Autodesk Fusion 360 part; units mm, degrees
note: some values were not read from the file. Set by a fixed rule: which sketch regions a step uses.
(part 2 of 2)
sketch "Standoffs" plane through (0, 4, 0) normal (0, 1, 0) x (-1, 0, 0)
  line L0 (-79.851, -68.7474) -> (-79.851, -61.1474)
  line L1 (-79.851, -61.1474) -> (-69.251, -61.1474)
  line L2 (-69.251, -61.1474) -> (-69.251, -68.7474)
  line L3 (-69.251, -68.7474) -> (-79.851, -68.7474)
  line L4 (-70.751, -3.7474) -> (-70.751, -11.3474)
  line L5 (-70.751, -11.3474) -> (-78.351, -11.3474)
  line L6 (-78.351, -11.3474) -> (-78.351, -3.7474)
  line L7 (-78.351, -3.7474) -> (-70.751, -3.7474)
  line L8 (-78.351, 49.0551) -> (-78.351, 56.6551)
  line L9 (-78.351, 56.6551) -> (-70.751, 56.6551)
  line L10 (-70.751, 56.6551) -> (-70.751, 49.0551)
  line L11 (-70.751, 49.0551) -> (-78.351, 49.0551)
  line L12 (-70.751, 11.3526) -> (-70.751, 3.7526)
  line L13 (-70.751, 3.7526) -> (-78.351, 3.7526)
  line L14 (-78.351, 3.7526) -> (-78.351, 11.3526)
  line L15 (-78.351, 11.3526) -> (-70.751, 11.3526)
  line L16 (-79.851, -55.1474) -> (-79.851, -47.5474)
  line L17 (-79.851, -47.5474) -> (-69.251, -47.5474)
  line L18 (-69.251, -47.5474) -> (-69.251, -55.1474)
  line L19 (-69.251, -55.1474) -> (-79.851, -55.1474)
  line L20 (-70.751, -18.8474) -> (-70.751, -26.4474)
  line L21 (-70.751, -26.4474) -> (-78.351, -26.4474)
  line L22 (-78.351, -26.4474) -> (-78.351, -18.8474)
  line L23 (-78.351, -18.8474) -> (-70.751, -18.8474)
  line L24 (-78.351, 33.9551) -> (-78.351, 41.5551)
  line L25 (-78.351, 41.5551) -> (-70.751, 41.5551)
  line L26 (-70.751, 41.5551) -> (-70.751, 33.9551)
  line L27 (-70.751, 33.9551) -> (-78.351, 33.9551)
  line L28 (-70.751, 26.4526) -> (-70.751, 18.8526)
  line L29 (-70.751, 18.8526) -> (-78.351, 18.8526)
  line L30 (-78.351, 18.8526) -> (-78.351, 26.4526)
  line L31 (-78.351, 26.4526) -> (-70.751, 26.4526)
  line L32 (-78.351, -41.5474) -> (-78.351, -33.9474)
  line L33 (-78.351, -33.9474) -> (-70.751, -33.9474)
  line L34 (-70.751, -33.9474) -> (-70.751, -41.5474)
  line L35 (-70.751, -41.5474) -> (-78.351, -41.5474)
  line L36 (-81.051, -86.395) -> (-68.051, -86.395)
  line L37 (-68.051, -86.395) -> (-68.051, 62.605)
  line L38 (-68.051, 62.605) -> (-81.051, 62.605)
  line L39 (-81.051, 62.605) -> (-81.051, -86.395)
  line L40 (-81.051, -42.5474) -> (-68.051, -42.5474)
  line L41 (-68.051, -42.5474) -> (-68.051, -46.5474)
  line L42 (-68.051, -46.5474) -> (-81.051, -46.5474)
  line L43 (-81.051, -46.5474) -> (-81.051, -42.5474)
  line L44 (-68.051, -56.1474) -> (-81.051, -56.1474)
  line L45 (-81.051, -56.1474) -> (-81.051, -60.1474)
  line L46 (-81.051, -60.1474) -> (-68.051, -60.1474)
  line L47 (-68.051, -60.1474) -> (-68.051, -56.1474)
  line L48 (-68.051, -69.7474) -> (-81.051, -69.7474)
  line L49 (-81.051, -69.7474) -> (-81.051, -74.7474)
  line L50 (-81.051, -74.7474) -> (-68.051, -74.7474)
  line L51 (-68.051, -74.7474) -> (-68.051, -69.7474)
  line L52 (-68.051, -32.9474) -> (-81.051, -32.9474)
  line L53 (-81.051, -32.9474) -> (-81.051, -27.4474)
  line L54 (-81.051, -27.4474) -> (-68.051, -27.4474)
  line L55 (-68.051, -27.4474) -> (-68.051, -32.9474)
  line L56 (-68.051, -17.8474) -> (-81.051, -17.8474)
  line L57 (-81.051, -17.8474) -> (-81.051, -12.3474)
  line L58 (-81.051, -12.3474) -> (-68.051, -12.3474)
  line L59 (-68.051, -12.3474) -> (-68.051, -17.8474)
  line L60 (-68.051, -2.7474) -> (-81.051, -2.7474)
  line L61 (-81.051, -2.7474) -> (-81.051, 2.7526)
  line L62 (-81.051, 2.7526) -> (-68.051, 2.7526)
  line L63 (-68.051, 2.7526) -> (-68.051, -2.7474)
  line L64 (-68.051, 12.3526) -> (-81.051, 12.3526)
  line L65 (-81.051, 12.3526) -> (-81.051, 17.8526)
  line L66 (-81.051, 17.8526) -> (-68.051, 17.8526)
  line L67 (-68.051, 17.8526) -> (-68.051, 12.3526)
  line L68 (-68.051, 27.4526) -> (-81.051, 27.4526)
  line L69 (-81.051, 27.4526) -> (-81.051, 32.9551)
  line L70 (-81.051, 32.9551) -> (-68.051, 32.9551)
  line L71 (-68.051, 32.9551) -> (-68.051, 27.4526)
  line L72 (-68.051, 42.5551) -> (-81.051, 42.5551)
  line L73 (-81.051, 42.5551) -> (-81.051, 48.0551)
  line L74 (-81.051, 48.0551) -> (-68.051, 48.0551)
  line L75 (-68.051, 48.0551) -> (-68.051, 42.5551)
  line L76 (-68.051, 57.6551) -> (-81.051, 57.6551)
  line L77 (-81.051, 57.6551) -> (-81.051, 62.605)
  line L78 (-81.051, 62.605) -> (-68.051, 62.605)
  line L79 (-68.051, 62.605) -> (-68.051, 57.6551)
  line L80 (-32.451, 96.755) -> (-27.151, 96.755)
  line L81 (-27.151, 96.755) -> (-27.151, 86.755)
  line L82 (-27.151, 86.755) -> (-32.451, 86.755)
  line L83 (-32.451, 86.755) -> (-32.451, 96.755)
  line L84 (-17.551, 96.755) -> (-12.251, 96.755)
  line L85 (-12.251, 96.755) -> (-12.251, 86.755)
  line L86 (-12.251, 86.755) -> (-17.551, 86.755)
  line L87 (-17.551, 86.755) -> (-17.551, 96.755)
  line L88 (-2.651, 96.755) -> (2.649, 96.755)
  line L89 (2.649, 96.755) -> (2.649, 86.755)
  line L90 (2.649, 86.755) -> (-2.651, 86.755)
  line L91 (-2.651, 86.755) -> (-2.651, 96.755)
  line L92 (12.249, 96.755) -> (17.549, 96.755)
  line L93 (17.549, 96.755) -> (17.549, 86.755)
  line L94 (17.549, 86.755) -> (12.249, 86.755)
  line L95 (12.249, 86.755) -> (12.249, 96.755)
  line L96 (27.149, 96.755) -> (32.451, 96.755)
  line L97 (32.451, 96.755) -> (32.451, 86.755)
  line L98 (32.451, 86.755) -> (27.149, 86.755)
  line L99 (27.149, 86.755) -> (27.149, 96.755)
  line L100 (68, 42.5551) -> (81, 42.5551)
  line L101 (81, 42.5551) -> (81, 47.5551)
  line L102 (81, 47.5551) -> (68, 47.5551)
  line L103 (68, 47.5551) -> (68, 42.5551)
  line L104 (81, 32.9551) -> (68, 32.9551)
  line L105 (68, 32.9551) -> (68, 27.4526)
  line L106 (68, 27.4526) -> (81, 27.4526)
  line L107 (81, 27.4526) -> (81, 32.9551)
  line L108 (81, 17.8526) -> (68, 17.8526)
  line L109 (68, 17.8526) -> (68, 12.3526)
  line L110 (68, 12.3526) -> (81, 12.3526)
  line L111 (81, 12.3526) -> (81, 17.8526)
  line L112 (68, 2.7526) -> (81, 2.7526)
  line L113 (81, 2.7526) -> (81, -2.7474)
  line L114 (81, -2.7474) -> (68, -2.7474)
  line L115 (68, -2.7474) -> (68, 2.7526)
  line L116 (81, -12.3474) -> (68, -12.3474)
  line L117 (68, -12.3474) -> (68, -17.8474)
  line L118 (68, -17.8474) -> (81, -17.8474)
  line L119 (81, -17.8474) -> (81, -12.3474)
  line L120 (81, -27.4474) -> (68, -27.4474)
  line L121 (68, -27.4474) -> (68, -32.9474)
  line L122 (68, -32.9474) -> (81, -32.9474)
  line L123 (81, -32.9474) -> (81, -27.4474)
  line L124 (81, -42.5474) -> (68, -42.5474)
  line L125 (68, -42.5474) -> (68, -46.5474)
  line L126 (68, -46.5474) -> (81, -46.5474)
  line L127 (81, -46.5474) -> (81, -42.5474)
  line L128 (81, -56.1474) -> (68, -56.1474)
  line L129 (68, -56.1474) -> (68, -60.1474)
  line L130 (68, -60.1474) -> (81, -60.1474)
  line L131 (81, -60.1474) -> (81, -56.1474)
  line L132 (81, -69.7474) -> (68, -69.7474)
  line L133 (68, -69.7474) -> (68, -74.7474)
  line L134 (68, -74.7474) -> (81, -74.7474)
  line L135 (81, -74.7474) -> (81, -69.7474)
  line L136 (42.051, -86.755) -> (46.051, -86.755)
  line L137 (46.051, -86.755) -> (46.051, -96.755)
  line L138 (46.051, -96.755) -> (42.051, -96.755)
  line L139 (42.051, -96.755) -> (42.051, -86.755)
  line L140 (27.149, -86.755) -> (32.451, -86.755)
  line L141 (32.451, -86.755) -> (32.451, -96.755)
  line L142 (32.451, -96.755) -> (27.149, -96.755)
  line L143 (27.149, -96.755) -> (27.149, -86.755)
  line L144 (12.249, -86.755) -> (17.549, -86.755)
  line L145 (17.549, -86.755) -> (17.549, -96.755)
  line L146 (17.549, -96.755) -> (12.249, -96.755)
  line L147 (12.249, -96.755) -> (12.249, -86.755)
  line L148 (-2.651, -86.755) -> (2.649, -86.755)
  line L149 (2.649, -86.755) -> (2.649, -96.755)
  line L150 (2.649, -96.755) -> (-2.651, -96.755)
  line L151 (-2.651, -96.755) -> (-2.651, -86.755)
  line L152 (-17.551, -86.755) -> (-12.251, -86.755)
  line L153 (-12.251, -86.755) -> (-12.251, -96.755)
  line L154 (-12.251, -96.755) -> (-17.551, -96.755)
  line L155 (-17.551, -96.755) -> (-17.551, -86.755)
  line L156 (-32.451, -86.755) -> (-27.151, -86.755)
  line L157 (-27.151, -86.755) -> (-27.151, -96.755)
  line L158 (-27.151, -96.755) -> (-32.451, -96.755)
  line L159 (-32.451, -96.755) -> (-32.451, -86.755)
  line L160 (-46.051, -86.755) -> (-42.051, -86.755)
  line L161 (-42.051, -86.755) -> (-42.051, -96.755)
  line L162 (-42.051, -96.755) -> (-46.051, -96.755)
  line L163 (-46.051, -96.755) -> (-46.051, -86.755)
  line L164 (-33.451, 95.555) -> (-33.451, 87.955)
  line L165 (-26.151, 87.955) -> (-26.151, 95.555)
  line L166 (42.499, 86.755) -> (-42.501, 86.755)
  line L167 (-42.501, 96.755) -> (42.499, 96.755)
  line L168 (18.549, 87.955) -> (18.549, 95.555)
  line L169 (11.249, 95.555) -> (11.249, 87.955)
  line L170 (3.649, 87.955) -> (3.649, 95.555)
  line L171 (-3.651, 95.555) -> (-3.651, 87.955)
  line L172 (-18.551, 95.555) -> (-18.551, 87.955)
  line L173 (-11.251, 87.955) -> (-11.251, 95.555)
  line L174 (26.149, 95.555) -> (26.149, 87.955)
  line L175 (33.451, 87.955) -> (33.451, 95.555)
  line L176 (70.751, 41.5551) -> (78.351, 41.5551)
  line L177 (70.751, 26.4526) -> (78.351, 26.4526)
  line L178 (78.351, 33.9551) -> (70.751, 33.9551)
  line L179 (78.351, 18.8526) -> (70.751, 18.8526)
  line L180 (70.751, 11.3526) -> (78.351, 11.3526)
  line L181 (78.351, 3.7526) -> (70.751, 3.7526)
  line L182 (70.751, -3.7474) -> (78.351, -3.7474)
  line L183 (78.351, -11.3474) -> (70.751, -11.3474)
  line L184 (70.751, -18.8474) -> (78.351, -18.8474)
  line L185 (78.351, -26.4474) -> (70.751, -26.4474)
  line L186 (70.751, -33.9474) -> (78.351, -33.9474)
  line L187 (78.351, -41.5474) -> (70.751, -41.5474)
  line L188 (69.251, -47.5474) -> (79.851, -47.5474)
  line L189 (79.851, -55.1474) -> (69.251, -55.1474)
  line L190 (69.251, -61.1474) -> (79.851, -61.1474)
  line L191 (79.851, -68.7474) -> (69.251, -68.7474)
  line L192 (-58.499, -86.755) -> (58.501, -86.755)
  line L193 (58.501, -96.755) -> (-58.499, -96.755)
  line L194 (47.051, -95.555) -> (47.051, -87.955)
  line L195 (41.051, -87.955) -> (41.051, -95.555)
  line L196 (33.451, -95.555) -> (33.451, -87.955)
  line L197 (26.149, -87.955) -> (26.149, -95.555)
  line L198 (18.549, -95.555) -> (18.549, -87.955)
  line L199 (11.249, -87.955) -> (11.249, -95.555)
  line L200 (-47.051, -87.955) -> (-47.051, -95.555)
  line L201 (-41.051, -95.555) -> (-41.051, -87.955)
  line L202 (-33.451, -87.955) -> (-33.451, -95.555)
  line L203 (-26.151, -95.555) -> (-26.151, -87.955)
  line L204 (-18.551, -87.955) -> (-18.551, -95.555)
  line L205 (-11.251, -95.555) -> (-11.251, -87.955)
  line L206 (-3.651, -87.955) -> (-3.651, -95.555)
  line L207 (3.649, -95.555) -> (3.649, -87.955)
  dimension "d304" = 1
  dimension "d305" = 5
  dimension "d306" = 1
  dimension "d307" = 1
  dimension "d308" = 1.2
  dimension "d309" = 1
  dimension "d310" = 1
  dimension "d311" = 1
  dimension "d312" = 1
  dimension "d313" = 1
  dimension "d314" = 1
  dimension "d315" = 1
  dimension "d316" = 1
  dimension "d317" = 1
  dimension "d318" = 1
  dimension "d319" = 1
  dimension "d320" = 1
  dimension "d321" = 1
  dimension "d322" = 1
  dimension "d323" = 1
  dimension "d324" = 1
  dimension "d325" = 1
  dimension "d326" = 1
  dimension "d327" = 1
  dimension "d328" = 1
  dimension "d329" = 1
  dimension "d330" = 1
  dimension "d331" = 1
  dimension "d332" = 7.6
  dimension "d333" = 1
  dimension "d334" = 1
  dimension "d335" = 1
  dimension "d336" = 5
  dimension "d337" = 1
  dimension "d338" = 1
  dimension "d339" = 1
  dimension "d340" = 1
  dimension "d341" = 1
  dimension "d342" = 1
  dimension "d343" = 1
  dimension "d344" = 1
  dimension "d345" = 1
  dimension "d346" = 1
  dimension "d347" = 5.5
  dimension "d348" = 1
  dimension "d349" = 1
  dimension "d350" = 1
  dimension "d351" = 1
  dimension "d352" = 1
  dimension "d353" = 5
  dimension "d354" = 1
  dimension "d355" = 1
  dimension "d356" = 1
  dimension "d357" = 1
  dimension "d358" = 1
  dimension "d359" = 1
  dimension "d360" = 1
  dimension "d361" = 1
  dimension "d362" = 1
  dimension "d363" = 1
  dimension "d364" = 1
  dimension "d365" = 1
  dimension "d366" = 1
  dimension "d367" = 1
  constraint horizontal L40
  constraint vertical L41
  constraint horizontal L42
  constraint vertical L43
  constraint coincident L37 L41.end
  constraint coincident L39 L40.start
  constraint horizontal L44
  constraint vertical L45
  constraint horizontal L46
  constraint vertical L47
  constraint coincident L39 L45.end
  constraint coincident L37 L44.start
  constraint horizontal L48
  constraint vertical L49
  constraint horizontal L50
  constraint vertical L51
  constraint coincident L39 L49.end
  constraint coincident L37 L48.start
  constraint horizontal L52
  constraint vertical L53
  constraint horizontal L54
  constraint vertical L55
  constraint coincident L39 L53.end
  constraint coincident L37 L52.start
  constraint horizontal L56
  constraint vertical L57
  constraint horizontal L58
  constraint vertical L59
  constraint coincident L37 L56.start
  constraint horizontal L60
  constraint vertical L61
  constraint horizontal L62
  constraint vertical L63
  constraint coincident L39 L61.end
  constraint coincident L37 L60.start
  constraint horizontal L64
  constraint vertical L65
  constraint horizontal L66
  constraint vertical L67
  constraint coincident L39 L65.end
  constraint coincident L37 L64.start
  constraint horizontal L68
  constraint vertical L69
  constraint horizontal L70
  constraint vertical L71
  constraint coincident L39 L69.end
  constraint coincident L37 L68.start
  constraint horizontal L72
  constraint vertical L73
  constraint horizontal L74
  constraint vertical L75
  constraint coincident L39 L73.end
  constraint coincident L37 L72.start
  constraint horizontal L76
  constraint vertical L77
  constraint horizontal L78
  constraint vertical L79
  constraint coincident L38.end L39.start
  constraint coincident L37 L76.start
  constraint horizontal L80
  constraint vertical L81
  constraint horizontal L82
  constraint vertical L83
  constraint horizontal L84
  constraint vertical L85
  constraint horizontal L86
  constraint vertical L87
  constraint horizontal L88
  constraint vertical L89
  constraint horizontal L90
  constraint vertical L91
  constraint horizontal L92
  constraint vertical L93
  constraint horizontal L94
  constraint vertical L95
  constraint horizontal L96
  constraint vertical L97
  constraint horizontal L98
  constraint vertical L99
  constraint horizontal L100
  constraint vertical L101
  constraint horizontal L102
  constraint vertical L103
  constraint horizontal L104
  constraint vertical L105
  constraint horizontal L106
  constraint vertical L107
  constraint horizontal L108
  constraint vertical L109
  constraint horizontal L110
  constraint vertical L111
  constraint horizontal L112
  constraint vertical L113
  constraint horizontal L114
  constraint vertical L115
  constraint horizontal L116
  constraint vertical L117
  constraint horizontal L118
  constraint vertical L119
  constraint horizontal L120
  constraint vertical L121
  constraint horizontal L122
  constraint vertical L123
  constraint horizontal L124
  constraint vertical L125
  constraint horizontal L126
  constraint vertical L127
  constraint horizontal L128
  constraint vertical L129
  constraint horizontal L130
  constraint vertical L131
  constraint horizontal L132
  constraint vertical L133
  constraint horizontal L134
  constraint vertical L135
  constraint horizontal L136
  constraint vertical L137
  constraint horizontal L138
  constraint vertical L139
  constraint horizontal L140
  constraint vertical L141
  constraint horizontal L142
  constraint vertical L143
  constraint horizontal L144
  constraint vertical L145
  constraint horizontal L146
  constraint vertical L147
  constraint horizontal L148
  constraint vertical L149
  constraint horizontal L150
  constraint vertical L151
  constraint horizontal L152
  constraint vertical L153
  constraint horizontal L154
  constraint vertical L155
  constraint horizontal L156
  constraint vertical L157
  constraint horizontal L158
  constraint vertical L159
  constraint horizontal L160
  constraint vertical L161
  constraint horizontal L162
  constraint vertical L163
  constraint collinear L82 L166
  constraint collinear L80 L167
  constraint collinear L84 L167
  constraint collinear L86 L166
  constraint collinear L90 L166
  constraint collinear L88 L167
  constraint collinear L92 L167
  constraint collinear L94 L166
  constraint collinear L98 L166
  constraint collinear L96 L167
  constraint collinear L136 L192
  constraint collinear L140 L192
  constraint collinear L146 L193
  constraint collinear L144 L192
  constraint collinear L142 L193
  constraint collinear L138 L193
  constraint collinear L148 L192
  constraint collinear L150 L193
  constraint collinear L154 L193
  constraint collinear L152 L192
  constraint collinear L156 L192
  constraint collinear L158 L193
  constraint collinear L162 L193
  constraint collinear L160 L192
  measures "d304" distance of L3 L48
  measures "d305" distance of L48 L50
  measures "d306" distance of L1 L46
  measures "d307" distance of L19 L44
  measures "d308" distance of L18 L37
  measures "d309" distance of L17 L42
  measures "d310" distance of L35 L40
  measures "d311" distance of L33 L52
  measures "d312" distance of L21 L54
  measures "d313" distance of L23 L56
  measures "d314" distance of L5 L58
  measures "d315" distance of L7 L60
  measures "d316" distance of L13 L62
  measures "d317" distance of L15 L64
  measures "d318" distance of L29 L66
  measures "d319" distance of L31 L68
  measures "d320" distance of L27 L70
  measures "d321" distance of L25 L72
  measures "d322" distance of L11 L74
  measures "d323" distance of L9 L76
  measures "d324" distance of L83 L164
  measures "d325" distance of L81 L165
  measures "d326" distance of L93 L168
  measures "d327" distance of L95 L169
  measures "d328" distance of L89 L170
  measures "d329" distance of L91 L171
  measures "d330" distance of L87 L172
  measures "d331" distance of L85 L173
  measures "d332" distance of L174.start L174.end
  measures "d333" distance of L99 L174
  measures "d334" distance of L97 L175
  measures "d335" distance of L100 L176
  measures "d336" distance of L100.end L101.end
  measures "d337" distance of L106 L177
  measures "d338" distance of L104 L178
  measures "d339" distance of L108 L179
  measures "d340" distance of L110 L180
  measures "d341" distance of L112 L181
  measures "d342" distance of L114 L182
  measures "d343" distance of L116 L183
  measures "d344" distance of L118 L184
  measures "d345" distance of L120 L185
  measures "d346" distance of L122 L186
  measures "d347" distance of L120.start L122.end
  measures "d348" distance of L124 L187
  measures "d349" distance of L126 L188
  measures "d350" distance of L128 L189
  measures "d351" distance of L130 L190
  measures "d352" distance of L132 L191
  measures "d353" distance of L132.start L134.end
  measures "d354" distance of L137 L194
  measures "d355" distance of L139 L195
  measures "d356" distance of L141 L196
  measures "d357" distance of L143 L197
  measures "d358" distance of L145 L198
  measures "d359" distance of L147 L199
  measures "d360" distance of L163 L200
  measures "d361" distance of L161 L201
  measures "d362" distance of L159 L202
  measures "d363" distance of L157 L203
  measures "d364" distance of L155 L204
  measures "d365" distance of L153 L205
  measures "d366" distance of L151 L206
  measures "d367" distance of L149 L207
extrude "Extrude7" add sketch "Standoffs" along normal blind 5.4 contours L37 L39 L48 L49 L50 L51 | L37 L39 L44 L45 L46 L47 | L37 L39 L40 L41 L42 L43 | L37 L39 L52 L53 L54 L55 | L37 L39 L56 L57 L58 L59 | L37 L39 L60 L61 L62 L63 | L37 L39 L64 L65 L66 L67 | L37 L39 L68 L69 L70 L71 | L37 L39 L72 L73 L74 L75 | L37 L38 L39 L76 L77 L78 L79
extrude "Extrude8" add sketch "Standoffs" along normal blind 5.4 contours L136 L137 L138 L139 L192 L193 | L140 L141 L142 L143 L192 L193 | L144 L145 L146 L147 L192 L193 | L148 L149 L150 L151 L192 L193 | L152 L153 L154 L155 L192 L193 | L156 L157 L158 L159 L192 L193 | L160 L161 L162 L163 L192 L193
extrude "Extrude9" add sketch "Standoffs" along normal blind 5.4 contours L100 L101 L102 L103 | L104 L105 L106 L107 | L108 L109 L110 L111 | L112 L113 L114 L115 | L116 L117 L118 L119 | L120 L121 L122 L123 | L124 L125 L126 L127 | L128 L129 L130 L131 | L132 L133 L134 L135
extrude "Extrude10" add sketch "Standoffs" along normal blind 5.4 contours L80 L81 L82 L83 L166 L167 | L84 L85 L86 L87 L166 L167 | L88 L89 L90 L91 L166 L167 | L92 L93 L94 L95 L166 L167 | L96 L97 L98 L99 L166 L167
sketch "Standoff Screw Holes" plane through (0, 9.4, 0) normal (0, 1, 0) x (-1, 0, 0)
  line L0 (27.149, 86.755) -> (32.451, 86.755)
  line L1 (32.451, 86.755) -> (32.451, 96.755)
  line L2 (32.451, 96.755) -> (27.149, 96.755)
  line L3 (27.149, 96.755) -> (27.149, 86.755)
  point P0 (74.5817, 45.2081)
  point P1 (74.5817, 30.1182)
  point P2 (74.5817, 15.2122)
  point P3 (74.5817, -0.0028)
  point P4 (74.5817, -15.1178)
  point P5 (74.5817, -30.2328)
  point P6 (74.5, -44.5)
named bodies: "Main Portrait Bezel"
